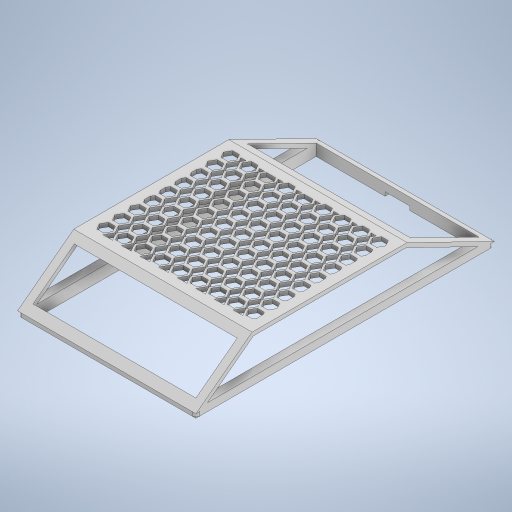
# Autodesk Inventor part: TopLid
Saved by Autodesk Inventor 2023.4 (Build 274418000, 418)
## iProperties
Created: 2026-02-22
Part Number: TopLid
Material: Generic
Document SubType Name: Modeling
Designer: 1017208
Density: 1 g/cm^3
Appearance: Default
Author: 1017208
## iProperties of the stored document TopLid_3DPrint.ipt
Created: 2026-02-22
Part Number: TopLid_3DPrint
Material: Generic
Document SubType Name: Modeling
Designer: 1017208
Density: 1 g/cm^3
Appearance: Default
Author: 1017208
Autodesk Inventor part; units mm, degrees
(part 1 of 2)
ref_plane "YZ Plane" through (0, 0, 0) normal (1, 0, 0) x (0, 1, 0)
ref_plane "XZ Plane" through (0, 0, 0) normal (0, 1, 0) x (-1, 0, 0)
ref_plane "XY Plane" through (0, 0, 0) normal (0, 0, 1) x (1, 0, 0)
sketch "Sketch1" plane through (0, 0, 0) normal (0, 1, 0) x (-1, 0, 0)
  line L0 (0, 0) -> (-139.7, 0)
  line L1 (-139.7, 0) -> (-139.7, -238.125)
  line L2 (-139.7, -238.125) -> (0, -238.125)
  line L3 (0, -238.125) -> (0, 0)
  line L4 (-3.175, -3.175) -> (-136.525, -3.175)
  line L5 (-136.525, -3.175) -> (-136.525, -234.95)
  line L6 (-136.525, -234.95) -> (-3.175, -234.95)
  line L7 (-3.175, -234.95) -> (-3.175, -3.175)
  line L8 (0, -238.125) -> (-139.7, -238.125)
  line L9 (-69.85, -238.125) -> (-69.85, -234.95)
  line L10 (-69.85, -238.125) -> (-59.69, -238.125)
  line L11 (-59.69, -238.125) -> (-80.01, -238.125)
  line L12 (-80.01, -238.125) -> (-80.01, -234.95)
  line L13 (-80.01, -234.95) -> (-59.69, -234.95)
  line L14 (-59.69, -234.95) -> (-59.69, -238.125)
  dimension "d0" = 139.7
  dimension "d1" = 238.125
  dimension "d2" = 3.175
  dimension "d3" = 10.16
  dimension "d4" = 20.32
  constraints: 30 end point, 7 equal length, 3 perpendicular, 2 horizontal, 2 midpoint, 2 point on line, 3 other
  measures "d0" distance of L2.end L1.end
  measures "d1" distance of L1.end L0.end
  measures "d2" distance between parallel lines of L3 L7
  measures "d3" distance of L9.start L10.end
  measures "d4" distance of L12.end L13.end
extrude "Extrusion1" add sketch "Sketch1" along normal blind 3.175 contours L3 L2 L14 L6 L7 L4 L5 L12 L1 L0
sketch "Sketch2" plane through (0, 3.175, 0) normal (0, 1, 0) x (1, 0, 0)
  line L0 (0, 238.125) -> (0, 0) projected
  line L1 (139.7, 238.125) -> (80.01, 238.125) projected
  line L2 (0, 0) -> (139.7, 0)
  line L3 (139.7, 0) -> (139.7, 238.125)
  line L4 (139.7, 238.125) -> (0, 238.125)
  line L5 (0, 238.125) -> (0, 0)
  line L6 (139.7, -3.175) -> (0, -3.175)
  line L7 (-3.175, 0) -> (-3.175, 238.125)
  line L8 (0, 241.3) -> (139.7, 241.3)
  line L9 (142.875, 238.125) -> (142.875, 0)
  arc A0 (0, 241.3) -> (-3.175, 238.125) centre (0, 238.125) ccw
  arc A1 (-3.175, 0) -> (0, -3.175) centre (0, 0) ccw
  arc A2 (139.7, -3.175) -> (142.875, 0) centre (139.7, 0) ccw
  arc A3 (142.875, 238.125) -> (139.7, 241.3) centre (139.7, 238.125) ccw
  dimension "d7" = 3.175
  constraints: 16 end point, 8 point on circle, 4 centre point, 4 coincident, 4 parallel, 3 tangent, 2 perpendicular, 1 horizontal
  measures "d7" distance between parallel lines of L2 L6
extrude "Extrusion2" add sketch "Sketch2" along normal blind 3.175 contours L4 L1 L3 L2 L0 | L6 A1 L7 A0 L8 A3 L9 A2
sketch "Sketch3" plane through (142.875, 3.175, 0) normal (1, 0, 0) x (0, 0, -1)
  line L0 (-3.175, 3.175) -> (241.3, 3.175)
  line L1 (0, 3.175) -> (238.125, 3.175) projected
  line L2 (119.0625, 3.175) -> (119.0625, 38.1)
  line L3 (119.0625, 38.1) -> (42.8625, 38.1)
  line L4 (119.0625, 38.1) -> (169.8625, 38.1)
  line L5 (-3.175, 3.175) -> (42.8625, 38.1)
  line L6 (169.8625, 38.1) -> (241.3, 3.175)
  line L7 (43.9305, 34.925) -> (119.0625, 34.925)
  line L8 (119.0625, 34.925) -> (169.1279, 34.925)
  line L9 (169.1279, 34.925) -> (227.5768, 6.35)
  line L10 (227.5768, 6.35) -> (6.2635, 6.35)
  line L11 (6.2635, 6.35) -> (43.9305, 34.925)
  point P0 (0, -3.175)
  dimension "d10" = 34.925
  dimension "d11" = 76.2
  dimension "d12" = 50.8
  dimension "d13" = 3.175
  constraints: 22 end point, 3 horizontal, 1 midpoint, 1 vertical, 4 other
  measures "d10" distance of L2.start L2.end
  measures "d11" distance of L2.end L3.end
  measures "d12" distance of L2.end L4.end
  measures "d13" distance between parallel lines of L3 L7
extrude "Extrusion3" add sketch "Sketch3" against normal blind 146.05 contours L5 L3 L2 L7 L11 L10 L0 | L2 L10 L9 L8 L4 L6 L0
sketch "Sketch4" plane through (0, 0, 0) normal (0, -1, 0) x (1, 0, 0)
  line L0 (0, 0) -> (139.7, 0) projected
  line L1 (0, -238.125) -> (139.7, -238.125) projected
  line L2 (0, 0) -> (139.7, 0)
  line L3 (139.7, 0) -> (139.7, -238.125)
  line L4 (139.7, -238.125) -> (0, -238.125)
  line L5 (0, -238.125) -> (0, 0)
  line L6 (136.525, -234.95) -> (136.525, -3.175)
  line L7 (136.525, -3.175) -> (3.175, -3.175)
  line L8 (3.175, -3.175) -> (3.175, -234.95)
  line L9 (3.175, -234.95) -> (136.525, -234.95)
  constraints: 16 end point, 4 parallel, 2 perpendicular, 1 horizontal, 3 other
extrude "Extrusion4" cut sketch "Sketch4" against normal blind 36.83 contours L9 L8 L7 L6
sketch "Sketch5" plane through (142.875, 41.275, -42.8625) normal (0, 1, 0) x (1, 0, 0)
  line L0 (-146.05, 127) -> (0, 127)
  line L1 (-3.6662, 6.35) -> (-149.7162, 6.35)
  line L2 (-149.7162, 6.35) -> (-146.05, 127)
  line L3 (-130.175, 122.2375) -> (-126.5088, 115.8875)
  line L4 (-126.5088, 115.8875) -> (-130.175, 109.5375)
  line L5 (-130.175, 109.5375) -> (-137.5073, 109.5375)
  line L6 (-137.5073, 109.5375) -> (-141.1735, 115.8875)
  line L7 (-141.1735, 115.8875) -> (-137.5073, 122.2375)
  line L8 (-137.5073, 122.2375) -> (-130.175, 122.2375)
  line L9 (-114.935, 122.2375) -> (-111.2688, 115.8875)
  line L10 (-111.2688, 115.8875) -> (-114.935, 109.5375)
  line L11 (-114.935, 109.5375) -> (-122.2673, 109.5375)
  line L12 (-122.2673, 109.5375) -> (-125.9335, 115.8875)
  line L13 (-125.9335, 115.8875) -> (-122.2673, 122.2375)
  line L14 (-122.2673, 122.2375) -> (-114.935, 122.2375)
  line L15 (-99.695, 122.2375) -> (-96.0288, 115.8875)
  line L16 (-96.0288, 115.8875) -> (-99.695, 109.5375)
  line L17 (-99.695, 109.5375) -> (-107.0273, 109.5375)
  line L18 (-107.0273, 109.5375) -> (-110.6935, 115.8875)
  line L19 (-110.6935, 115.8875) -> (-107.0273, 122.2375)
  line L20 (-107.0273, 122.2375) -> (-99.695, 122.2375)
  line L21 (-84.455, 122.2375) -> (-80.7888, 115.8875)
  line L22 (-80.7888, 115.8875) -> (-84.455, 109.5375)
  line L23 (-84.455, 109.5375) -> (-91.7873, 109.5375)
  line L24 (-91.7873, 109.5375) -> (-95.4535, 115.8875)
  line L25 (-95.4535, 115.8875) -> (-91.7873, 122.2375)
  line L26 (-91.7873, 122.2375) -> (-84.455, 122.2375)
  line L27 (-69.215, 122.2375) -> (-65.5488, 115.8875)
  line L28 (-65.5488, 115.8875) -> (-69.215, 109.5375)
  line L29 (-69.215, 109.5375) -> (-76.5473, 109.5375)
  line L30 (-76.5473, 109.5375) -> (-80.2135, 115.8875)
  line L31 (-80.2135, 115.8875) -> (-76.5473, 122.2375)
  line L32 (-76.5473, 122.2375) -> (-69.215, 122.2375)
  line L33 (-53.975, 122.2375) -> (-50.3088, 115.8875)
  line L34 (-50.3088, 115.8875) -> (-53.975, 109.5375)
  line L35 (-53.975, 109.5375) -> (-61.3073, 109.5375)
  line L36 (-61.3073, 109.5375) -> (-64.9735, 115.8875)
  line L37 (-64.9735, 115.8875) -> (-61.3073, 122.2375)
  line L38 (-61.3073, 122.2375) -> (-53.975, 122.2375)
  line L39 (-38.735, 122.2375) -> (-35.0688, 115.8875)
  line L40 (-35.0688, 115.8875) -> (-38.735, 109.5375)
  line L41 (-38.735, 109.5375) -> (-46.0673, 109.5375)
  line L42 (-46.0673, 109.5375) -> (-49.7335, 115.8875)
  line L43 (-49.7335, 115.8875) -> (-46.0673, 122.2375)
  line L44 (-46.0673, 122.2375) -> (-38.735, 122.2375)
  line L45 (-23.495, 122.2375) -> (-19.8288, 115.8875)
  line L46 (-19.8288, 115.8875) -> (-23.495, 109.5375)
  line L47 (-23.495, 109.5375) -> (-30.8273, 109.5375)
  line L48 (-30.8273, 109.5375) -> (-34.4935, 115.8875)
  line L49 (-34.4935, 115.8875) -> (-30.8273, 122.2375)
  line L50 (-30.8273, 122.2375) -> (-23.495, 122.2375)
  line L51 (-8.255, 122.2375) -> (-4.5888, 115.8875)
  line L52 (-4.5888, 115.8875) -> (-8.255, 109.5375)
  line L53 (-8.255, 109.5375) -> (-15.5873, 109.5375)
  line L54 (-15.5873, 109.5375) -> (-19.2535, 115.8875)
  line L55 (-19.2535, 115.8875) -> (-15.5873, 122.2375)
  line L56 (-15.5873, 122.2375) -> (-8.255, 122.2375)
  line L57 (-130.175, 109.5375) -> (-126.5088, 103.1875)
  line L58 (-126.5088, 103.1875) -> (-130.175, 96.8375)
  line L59 (-130.175, 96.8375) -> (-137.5073, 96.8375)
  line L60 (-137.5073, 96.8375) -> (-141.1735, 103.1875)
  line L61 (-141.1735, 103.1875) -> (-137.5073, 109.5375)
  line L62 (-137.5073, 109.5375) -> (-130.175, 109.5375)
  line L63 (-114.935, 109.5375) -> (-111.2688, 103.1875)
  line L64 (-111.2688, 103.1875) -> (-114.935, 96.8375)
  line L65 (-114.935, 96.8375) -> (-122.2673, 96.8375)
  line L66 (-122.2673, 96.8375) -> (-125.9335, 103.1875)
  line L67 (-125.9335, 103.1875) -> (-122.2673, 109.5375)
  line L68 (-122.2673, 109.5375) -> (-114.935, 109.5375)
  line L69 (-99.695, 109.5375) -> (-96.0288, 103.1875)
  line L70 (-96.0288, 103.1875) -> (-99.695, 96.8375)
  line L71 (-99.695, 96.8375) -> (-107.0273, 96.8375)
  line L72 (-107.0273, 96.8375) -> (-110.6935, 103.1875)
  line L73 (-110.6935, 103.1875) -> (-107.0273, 109.5375)
  line L74 (-107.0273, 109.5375) -> (-99.695, 109.5375)
  line L75 (-84.455, 109.5375) -> (-80.7888, 103.1875)
  line L76 (-80.7888, 103.1875) -> (-84.455, 96.8375)
  line L77 (-84.455, 96.8375) -> (-91.7873, 96.8375)
  line L78 (-91.7873, 96.8375) -> (-95.4535, 103.1875)
  line L79 (-95.4535, 103.1875) -> (-91.7873, 109.5375)
  line L80 (-91.7873, 109.5375) -> (-84.455, 109.5375)
  line L81 (-69.215, 109.5375) -> (-65.5488, 103.1875)
  line L82 (-65.5488, 103.1875) -> (-69.215, 96.8375)
  line L83 (-69.215, 96.8375) -> (-76.5473, 96.8375)
  line L84 (-76.5473, 96.8375) -> (-80.2135, 103.1875)
  line L85 (-80.2135, 103.1875) -> (-76.5473, 109.5375)
  line L86 (-76.5473, 109.5375) -> (-69.215, 109.5375)
  line L87 (-53.975, 109.5375) -> (-50.3088, 103.1875)
  line L88 (-50.3088, 103.1875) -> (-53.975, 96.8375)
  line L89 (-53.975, 96.8375) -> (-61.3073, 96.8375)
  line L90 (-61.3073, 96.8375) -> (-64.9735, 103.1875)
  line L91 (-64.9735, 103.1875) -> (-61.3073, 109.5375)
  line L92 (-61.3073, 109.5375) -> (-53.975, 109.5375)
  line L93 (-38.735, 109.5375) -> (-35.0688, 103.1875)
  line L94 (-35.0688, 103.1875) -> (-38.735, 96.8375)
  line L95 (-38.735, 96.8375) -> (-46.0673, 96.8375)
  line L96 (-46.0673, 96.8375) -> (-49.7335, 103.1875)
  line L97 (-49.7335, 103.1875) -> (-46.0673, 109.5375)
  line L98 (-46.0673, 109.5375) -> (-38.735, 109.5375)
  line L99 (-23.495, 109.5375) -> (-19.8288, 103.1875)
  line L100 (-19.8288, 103.1875) -> (-23.495, 96.8375)
  line L101 (-23.495, 96.8375) -> (-30.8273, 96.8375)
  line L102 (-30.8273, 96.8375) -> (-34.4935, 103.1875)
  line L103 (-34.4935, 103.1875) -> (-30.8273, 109.5375)
  line L104 (-30.8273, 109.5375) -> (-23.495, 109.5375)
  line L105 (-8.255, 109.5375) -> (-4.5888, 103.1875)
  line L106 (-4.5888, 103.1875) -> (-8.255, 96.8375)
  line L107 (-8.255, 96.8375) -> (-15.5873, 96.8375)
  line L108 (-15.5873, 96.8375) -> (-19.2535, 103.1875)
  line L109 (-19.2535, 103.1875) -> (-15.5873, 109.5375)
  line L110 (-15.5873, 109.5375) -> (-8.255, 109.5375)
  line L111 (-130.175, 96.8375) -> (-126.5088, 90.4875)
  line L112 (-126.5088, 90.4875) -> (-130.175, 84.1375)
  line L113 (-130.175, 84.1375) -> (-137.5073, 84.1375)
  line L114 (-137.5073, 84.1375) -> (-141.1735, 90.4875)
  line L115 (-141.1735, 90.4875) -> (-137.5073, 96.8375)
  line L116 (-137.5073, 96.8375) -> (-130.175, 96.8375)
  line L117 (-114.935, 96.8375) -> (-111.2688, 90.4875)
  line L118 (-111.2688, 90.4875) -> (-114.935, 84.1375)
  line L119 (-114.935, 84.1375) -> (-122.2673, 84.1375)
  line L120 (-122.2673, 84.1375) -> (-125.9335, 90.4875)
  line L121 (-125.9335, 90.4875) -> (-122.2673, 96.8375)
  line L122 (-122.2673, 96.8375) -> (-114.935, 96.8375)
  line L123 (-99.695, 96.8375) -> (-96.0288, 90.4875)
  line L124 (-96.0288, 90.4875) -> (-99.695, 84.1375)
  line L125 (-99.695, 84.1375) -> (-107.0273, 84.1375)
  line L126 (-107.0273, 84.1375) -> (-110.6935, 90.4875)
  line L127 (-110.6935, 90.4875) -> (-107.0273, 96.8375)
  line L128 (-107.0273, 96.8375) -> (-99.695, 96.8375)
  line L129 (-84.455, 96.8375) -> (-80.7888, 90.4875)
  line L130 (-80.7888, 90.4875) -> (-84.455, 84.1375)
  line L131 (-84.455, 84.1375) -> (-91.7873, 84.1375)
  line L132 (-91.7873, 84.1375) -> (-95.4535, 90.4875)
  line L133 (-95.4535, 90.4875) -> (-91.7873, 96.8375)
  line L134 (-91.7873, 96.8375) -> (-84.455, 96.8375)
  line L135 (-69.215, 96.8375) -> (-65.5488, 90.4875)
  line L136 (-65.5488, 90.4875) -> (-69.215, 84.1375)
  line L137 (-69.215, 84.1375) -> (-76.5473, 84.1375)
  line L138 (-76.5473, 84.1375) -> (-80.2135, 90.4875)
  line L139 (-80.2135, 90.4875) -> (-76.5473, 96.8375)
  line L140 (-76.5473, 96.8375) -> (-69.215, 96.8375)
  line L141 (-53.975, 96.8375) -> (-50.3088, 90.4875)
  line L142 (-50.3088, 90.4875) -> (-53.975, 84.1375)
  line L143 (-53.975, 84.1375) -> (-61.3073, 84.1375)
  line L144 (-61.3073, 84.1375) -> (-64.9735, 90.4875)
  line L145 (-64.9735, 90.4875) -> (-61.3073, 96.8375)
  line L146 (-61.3073, 96.8375) -> (-53.975, 96.8375)
  line L147 (-38.735, 96.8375) -> (-35.0688, 90.4875)
  line L148 (-35.0688, 90.4875) -> (-38.735, 84.1375)
  line L149 (-38.735, 84.1375) -> (-46.0673, 84.1375)
  line L150 (-46.0673, 84.1375) -> (-49.7335, 90.4875)
  line L151 (-49.7335, 90.4875) -> (-46.0673, 96.8375)
  line L152 (-46.0673, 96.8375) -> (-38.735, 96.8375)
  line L153 (-23.495, 96.8375) -> (-19.8288, 90.4875)
  line L154 (-19.8288, 90.4875) -> (-23.495, 84.1375)
  line L155 (-23.495, 84.1375) -> (-30.8273, 84.1375)
  line L156 (-30.8273, 84.1375) -> (-34.4935, 90.4875)
  line L157 (-34.4935, 90.4875) -> (-30.8273, 96.8375)
  line L158 (-30.8273, 96.8375) -> (-23.495, 96.8375)
  line L159 (-8.255, 96.8375) -> (-4.5888, 90.4875)
  line L160 (-4.5888, 90.4875) -> (-8.255, 84.1375)
  line L161 (-8.255, 84.1375) -> (-15.5873, 84.1375)
  line L162 (-15.5873, 84.1375) -> (-19.2535, 90.4875)
  line L163 (-19.2535, 90.4875) -> (-15.5873, 96.8375)
  line L164 (-15.5873, 96.8375) -> (-8.255, 96.8375)
  line L165 (-130.175, 84.1375) -> (-126.5088, 77.7875)
  line L166 (-126.5088, 77.7875) -> (-130.175, 71.4375)
  line L167 (-130.175, 71.4375) -> (-137.5073, 71.4375)
  line L168 (-137.5073, 71.4375) -> (-141.1735, 77.7875)
  line L169 (-141.1735, 77.7875) -> (-137.5073, 84.1375)
  line L170 (-137.5073, 84.1375) -> (-130.175, 84.1375)
  line L171 (-114.935, 84.1375) -> (-111.2688, 77.7875)
  line L172 (-111.2688, 77.7875) -> (-114.935, 71.4375)
  line L173 (-114.935, 71.4375) -> (-122.2673, 71.4375)
  line L174 (-122.2673, 71.4375) -> (-125.9335, 77.7875)
  line L175 (-125.9335, 77.7875) -> (-122.2673, 84.1375)
  line L176 (-122.2673, 84.1375) -> (-114.935, 84.1375)
  line L177 (-99.695, 84.1375) -> (-96.0288, 77.7875)
  line L178 (-96.0288, 77.7875) -> (-99.695, 71.4375)
  line L179 (-99.695, 71.4375) -> (-107.0273, 71.4375)
  line L180 (-107.0273, 71.4375) -> (-110.6935, 77.7875)
  line L181 (-110.6935, 77.7875) -> (-107.0273, 84.1375)
  line L182 (-107.0273, 84.1375) -> (-99.695, 84.1375)
  line L183 (-84.455, 84.1375) -> (-80.7888, 77.7875)
  line L184 (-80.7888, 77.7875) -> (-84.455, 71.4375)
  line L185 (-84.455, 71.4375) -> (-91.7873, 71.4375)
  line L186 (-91.7873, 71.4375) -> (-95.4535, 77.7875)
  line L187 (-95.4535, 77.7875) -> (-91.7873, 84.1375)
  line L188 (-91.7873, 84.1375) -> (-84.455, 84.1375)
  line L189 (-69.215, 84.1375) -> (-65.5488, 77.7875)
  line L190 (-65.5488, 77.7875) -> (-69.215, 71.4375)
  line L191 (-69.215, 71.4375) -> (-76.5473, 71.4375)
  line L192 (-76.5473, 71.4375) -> (-80.2135, 77.7875)
  line L193 (-80.2135, 77.7875) -> (-76.5473, 84.1375)
  line L194 (-76.5473, 84.1375) -> (-69.215, 84.1375)
  line L195 (-53.975, 84.1375) -> (-50.3088, 77.7875)
  line L196 (-50.3088, 77.7875) -> (-53.975, 71.4375)
  line L197 (-53.975, 71.4375) -> (-61.3073, 71.4375)
  line L198 (-61.3073, 71.4375) -> (-64.9735, 77.7875)
  line L199 (-64.9735, 77.7875) -> (-61.3073, 84.1375)
  line L200 (-61.3073, 84.1375) -> (-53.975, 84.1375)
  line L201 (-38.735, 84.1375) -> (-35.0688, 77.7875)
  line L202 (-35.0688, 77.7875) -> (-38.735, 71.4375)
  line L203 (-38.735, 71.4375) -> (-46.0673, 71.4375)
  line L204 (-46.0673, 71.4375) -> (-49.7335, 77.7875)
  line L205 (-49.7335, 77.7875) -> (-46.0673, 84.1375)
  line L206 (-46.0673, 84.1375) -> (-38.735, 84.1375)
  line L207 (-23.495, 84.1375) -> (-19.8288, 77.7875)
  line L208 (-19.8288, 77.7875) -> (-23.495, 71.4375)
  line L209 (-23.495, 71.4375) -> (-30.8273, 71.4375)
  line L210 (-30.8273, 71.4375) -> (-34.4935, 77.7875)
  line L211 (-34.4935, 77.7875) -> (-30.8273, 84.1375)
  line L212 (-30.8273, 84.1375) -> (-23.495, 84.1375)
  line L213 (-8.255, 84.1375) -> (-4.5888, 77.7875)
  line L214 (-4.5888, 77.7875) -> (-8.255, 71.4375)
  line L215 (-8.255, 71.4375) -> (-15.5873, 71.4375)
  line L216 (-15.5873, 71.4375) -> (-19.2535, 77.7875)
  line L217 (-19.2535, 77.7875) -> (-15.5873, 84.1375)
  line L218 (-15.5873, 84.1375) -> (-8.255, 84.1375)
  line L219 (-130.175, 71.4375) -> (-126.5088, 65.0875)
  line L220 (-126.5088, 65.0875) -> (-130.175, 58.7375)
  line L221 (-130.175, 58.7375) -> (-137.5073, 58.7375)
  line L222 (-137.5073, 58.7375) -> (-141.1735, 65.0875)
  line L223 (-141.1735, 65.0875) -> (-137.5073, 71.4375)
  line L224 (-137.5073, 71.4375) -> (-130.175, 71.4375)
  line L225 (-114.935, 71.4375) -> (-111.2688, 65.0875)
  line L226 (-111.2688, 65.0875) -> (-114.935, 58.7375)
  line L227 (-114.935, 58.7375) -> (-122.2673, 58.7375)
  line L228 (-122.2673, 58.7375) -> (-125.9335, 65.0875)
  line L229 (-125.9335, 65.0875) -> (-122.2673, 71.4375)
  line L230 (-122.2673, 71.4375) -> (-114.935, 71.4375)
  line L231 (-99.695, 71.4375) -> (-96.0288, 65.0875)
  line L232 (-96.0288, 65.0875) -> (-99.695, 58.7375)
  line L233 (-99.695, 58.7375) -> (-107.0273, 58.7375)
  line L234 (-107.0273, 58.7375) -> (-110.6935, 65.0875)
  line L235 (-110.6935, 65.0875) -> (-107.0273, 71.4375)
  line L236 (-107.0273, 71.4375) -> (-99.695, 71.4375)
  line L237 (-84.455, 71.4375) -> (-80.7888, 65.0875)
  line L238 (-80.7888, 65.0875) -> (-84.455, 58.7375)
  line L239 (-84.455, 58.7375) -> (-91.7873, 58.7375)
  line L240 (-91.7873, 58.7375) -> (-95.4535, 65.0875)
  line L241 (-95.4535, 65.0875) -> (-91.7873, 71.4375)
  line L242 (-91.7873, 71.4375) -> (-84.455, 71.4375)
  line L243 (-69.215, 71.4375) -> (-65.5488, 65.0875)
  line L244 (-65.5488, 65.0875) -> (-69.215, 58.7375)
  line L245 (-69.215, 58.7375) -> (-76.5473, 58.7375)
  line L246 (-76.5473, 58.7375) -> (-80.2135, 65.0875)
  line L247 (-80.2135, 65.0875) -> (-76.5473, 71.4375)
  line L248 (-76.5473, 71.4375) -> (-69.215, 71.4375)
  line L249 (-53.975, 71.4375) -> (-50.3088, 65.0875)
  line L250 (-50.3088, 65.0875) -> (-53.975, 58.7375)
  line L251 (-53.975, 58.7375) -> (-61.3073, 58.7375)
  line L252 (-61.3073, 58.7375) -> (-64.9735, 65.0875)
  line L253 (-64.9735, 65.0875) -> (-61.3073, 71.4375)
  line L254 (-61.3073, 71.4375) -> (-53.975, 71.4375)
  line L255 (-38.735, 71.4375) -> (-35.0688, 65.0875)
  line L256 (-35.0688, 65.0875) -> (-38.735, 58.7375)
  line L257 (-38.735, 58.7375) -> (-46.0673, 58.7375)
  line L258 (-46.0673, 58.7375) -> (-49.7335, 65.0875)
  line L259 (-49.7335, 65.0875) -> (-46.0673, 71.4375)
  line L260 (-46.0673, 71.4375) -> (-38.735, 71.4375)
  line L261 (-23.495, 71.4375) -> (-19.8288, 65.0875)
  line L262 (-19.8288, 65.0875) -> (-23.495, 58.7375)
  line L263 (-23.495, 58.7375) -> (-30.8273, 58.7375)
  line L264 (-30.8273, 58.7375) -> (-34.4935, 65.0875)
  line L265 (-34.4935, 65.0875) -> (-30.8273, 71.4375)
  line L266 (-30.8273, 71.4375) -> (-23.495, 71.4375)
  line L267 (-8.255, 71.4375) -> (-4.5888, 65.0875)
  line L268 (-4.5888, 65.0875) -> (-8.255, 58.7375)
  line L269 (-8.255, 58.7375) -> (-15.5873, 58.7375)
  line L270 (-15.5873, 58.7375) -> (-19.2535, 65.0875)
  line L271 (-19.2535, 65.0875) -> (-15.5873, 71.4375)
  line L272 (-15.5873, 71.4375) -> (-8.255, 71.4375)
  line L273 (-130.175, 58.7375) -> (-126.5088, 52.3875)
  line L274 (-126.5088, 52.3875) -> (-130.175, 46.0375)
  line L275 (-130.175, 46.0375) -> (-137.5073, 46.0375)
  line L276 (-137.5073, 46.0375) -> (-141.1735, 52.3875)
  line L277 (-141.1735, 52.3875) -> (-137.5073, 58.7375)
  line L278 (-137.5073, 58.7375) -> (-130.175, 58.7375)
  line L279 (-114.935, 58.7375) -> (-111.2688, 52.3875)
  line L280 (-111.2688, 52.3875) -> (-114.935, 46.0375)
  line L281 (-114.935, 46.0375) -> (-122.2673, 46.0375)
  line L282 (-122.2673, 46.0375) -> (-125.9335, 52.3875)
  line L283 (-125.9335, 52.3875) -> (-122.2673, 58.7375)
  line L284 (-122.2673, 58.7375) -> (-114.935, 58.7375)
  line L285 (-99.695, 58.7375) -> (-96.0288, 52.3875)
  line L286 (-96.0288, 52.3875) -> (-99.695, 46.0375)
  line L287 (-99.695, 46.0375) -> (-107.0273, 46.0375)
  line L288 (-107.0273, 46.0375) -> (-110.6935, 52.3875)
  line L289 (-110.6935, 52.3875) -> (-107.0273, 58.7375)
  line L290 (-107.0273, 58.7375) -> (-99.695, 58.7375)
  line L291 (-84.455, 58.7375) -> (-80.7888, 52.3875)
  line L292 (-80.7888, 52.3875) -> (-84.455, 46.0375)
  line L293 (-84.455, 46.0375) -> (-91.7873, 46.0375)
  line L294 (-91.7873, 46.0375) -> (-95.4535, 52.3875)
  line L295 (-95.4535, 52.3875) -> (-91.7873, 58.7375)
  line L296 (-91.7873, 58.7375) -> (-84.455, 58.7375)
  line L297 (-69.215, 58.7375) -> (-65.5488, 52.3875)
  line L298 (-65.5488, 52.3875) -> (-69.215, 46.0375)
  line L299 (-69.215, 46.0375) -> (-76.5473, 46.0375)
  line L300 (-76.5473, 46.0375) -> (-80.2135, 52.3875)
  line L301 (-80.2135, 52.3875) -> (-76.5473, 58.7375)
  line L302 (-76.5473, 58.7375) -> (-69.215, 58.7375)
  line L303 (-53.975, 58.7375) -> (-50.3088, 52.3875)
  line L304 (-50.3088, 52.3875) -> (-53.975, 46.0375)
  line L305 (-53.975, 46.0375) -> (-61.3073, 46.0375)
  line L306 (-61.3073, 46.0375) -> (-64.9735, 52.3875)
  line L307 (-64.9735, 52.3875) -> (-61.3073, 58.7375)
  line L308 (-61.3073, 58.7375) -> (-53.975, 58.7375)
  line L309 (-38.735, 58.7375) -> (-35.0688, 52.3875)
  line L310 (-35.0688, 52.3875) -> (-38.735, 46.0375)
  line L311 (-38.735, 46.0375) -> (-46.0673, 46.0375)
  line L312 (-46.0673, 46.0375) -> (-49.7335, 52.3875)
  line L313 (-49.7335, 52.3875) -> (-46.0673, 58.7375)
  line L314 (-46.0673, 58.7375) -> (-38.735, 58.7375)
  line L315 (-23.495, 58.7375) -> (-19.8288, 52.3875)
  line L316 (-19.8288, 52.3875) -> (-23.495, 46.0375)
  line L317 (-23.495, 46.0375) -> (-30.8273, 46.0375)
  line L318 (-30.8273, 46.0375) -> (-34.4935, 52.3875)
  line L319 (-34.4935, 52.3875) -> (-30.8273, 58.7375)
  line L320 (-30.8273, 58.7375) -> (-23.495, 58.7375)
  line L321 (-8.255, 58.7375) -> (-4.5888, 52.3875)
  line L322 (-4.5888, 52.3875) -> (-8.255, 46.0375)
  line L323 (-8.255, 46.0375) -> (-15.5873, 46.0375)
  line L324 (-15.5873, 46.0375) -> (-19.2535, 52.3875)
  line L325 (-19.2535, 52.3875) -> (-15.5873, 58.7375)
  line L326 (-15.5873, 58.7375) -> (-8.255, 58.7375)
  line L327 (-130.175, 46.0375) -> (-126.5088, 39.6875)
  line L328 (-126.5088, 39.6875) -> (-130.175, 33.3375)
  line L329 (-130.175, 33.3375) -> (-137.5073, 33.3375)
  line L330 (-137.5073, 33.3375) -> (-141.1735, 39.6875)
  line L331 (-141.1735, 39.6875) -> (-137.5073, 46.0375)
  line L332 (-137.5073, 46.0375) -> (-130.175, 46.0375)
  line L333 (-114.935, 46.0375) -> (-111.2688, 39.6875)
  line L334 (-111.2688, 39.6875) -> (-114.935, 33.3375)
  line L335 (-114.935, 33.3375) -> (-122.2673, 33.3375)
  line L336 (-122.2673, 33.3375) -> (-125.9335, 39.6875)
  line L337 (-125.9335, 39.6875) -> (-122.2673, 46.0375)
  line L338 (-122.2673, 46.0375) -> (-114.935, 46.0375)
  line L339 (-99.695, 46.0375) -> (-96.0288, 39.6875)
  line L340 (-96.0288, 39.6875) -> (-99.695, 33.3375)
  line L341 (-99.695, 33.3375) -> (-107.0273, 33.3375)
  line L342 (-107.0273, 33.3375) -> (-110.6935, 39.6875)
  line L343 (-110.6935, 39.6875) -> (-107.0273, 46.0375)
  line L344 (-107.0273, 46.0375) -> (-99.695, 46.0375)
  line L345 (-84.455, 46.0375) -> (-80.7888, 39.6875)
  line L346 (-80.7888, 39.6875) -> (-84.455, 33.3375)
  line L347 (-84.455, 33.3375) -> (-91.7873, 33.3375)
  line L348 (-91.7873, 33.3375) -> (-95.4535, 39.6875)
  line L349 (-95.4535, 39.6875) -> (-91.7873, 46.0375)
  line L350 (-91.7873, 46.0375) -> (-84.455, 46.0375)
  line L351 (-69.215, 46.0375) -> (-65.5488, 39.6875)
  line L352 (-65.5488, 39.6875) -> (-69.215, 33.3375)
  line L353 (-69.215, 33.3375) -> (-76.5473, 33.3375)
  line L354 (-76.5473, 33.3375) -> (-80.2135, 39.6875)
  line L355 (-80.2135, 39.6875) -> (-76.5473, 46.0375)
  line L356 (-76.5473, 46.0375) -> (-69.215, 46.0375)
  line L357 (-53.975, 46.0375) -> (-50.3088, 39.6875)
  line L358 (-50.3088, 39.6875) -> (-53.975, 33.3375)
  line L359 (-53.975, 33.3375) -> (-61.3073, 33.3375)
  line L360 (-61.3073, 33.3375) -> (-64.9735, 39.6875)
  line L361 (-64.9735, 39.6875) -> (-61.3073, 46.0375)
  line L362 (-61.3073, 46.0375) -> (-53.975, 46.0375)
  line L363 (-38.735, 46.0375) -> (-35.0688, 39.6875)
  line L364 (-35.0688, 39.6875) -> (-38.735, 33.3375)
  line L365 (-38.735, 33.3375) -> (-46.0673, 33.3375)
  line L366 (-46.0673, 33.3375) -> (-49.7335, 39.6875)
  line L367 (-49.7335, 39.6875) -> (-46.0673, 46.0375)
  line L368 (-46.0673, 46.0375) -> (-38.735, 46.0375)
  line L369 (-23.495, 46.0375) -> (-19.8288, 39.6875)
  line L370 (-19.8288, 39.6875) -> (-23.495, 33.3375)
  line L371 (-23.495, 33.3375) -> (-30.8273, 33.3375)
  line L372 (-30.8273, 33.3375) -> (-34.4935, 39.6875)
  line L373 (-34.4935, 39.6875) -> (-30.8273, 46.0375)
  line L374 (-30.8273, 46.0375) -> (-23.495, 46.0375)
  line L375 (-8.255, 46.0375) -> (-4.5888, 39.6875)
  line L376 (-4.5888, 39.6875) -> (-8.255, 33.3375)
  line L377 (-8.255, 33.3375) -> (-15.5873, 33.3375)
  line L378 (-15.5873, 33.3375) -> (-19.2535, 39.6875)
  line L379 (-19.2535, 39.6875) -> (-15.5873, 46.0375)
  line L380 (-15.5873, 46.0375) -> (-8.255, 46.0375)
  line L381 (-130.175, 33.3375) -> (-126.5088, 26.9875)
  line L382 (-126.5088, 26.9875) -> (-130.175, 20.6375)
  line L383 (-130.175, 20.6375) -> (-137.5073, 20.6375)
  line L384 (-137.5073, 20.6375) -> (-141.1735, 26.9875)
  line L385 (-141.1735, 26.9875) -> (-137.5073, 33.3375)
  line L386 (-137.5073, 33.3375) -> (-130.175, 33.3375)
  line L387 (-114.935, 33.3375) -> (-111.2688, 26.9875)
  line L388 (-111.2688, 26.9875) -> (-114.935, 20.6375)
  line L389 (-114.935, 20.6375) -> (-122.2673, 20.6375)
  line L390 (-122.2673, 20.6375) -> (-125.9335, 26.9875)
  line L391 (-125.9335, 26.9875) -> (-122.2673, 33.3375)
  line L392 (-122.2673, 33.3375) -> (-114.935, 33.3375)
  line L393 (-99.695, 33.3375) -> (-96.0288, 26.9875)
  line L394 (-96.0288, 26.9875) -> (-99.695, 20.6375)
  line L395 (-99.695, 20.6375) -> (-107.0273, 20.6375)
  line L396 (-107.0273, 20.6375) -> (-110.6935, 26.9875)
  line L397 (-110.6935, 26.9875) -> (-107.0273, 33.3375)
  line L398 (-107.0273, 33.3375) -> (-99.695, 33.3375)
  line L399 (-84.455, 33.3375) -> (-80.7888, 26.9875)
  line L400 (-80.7888, 26.9875) -> (-84.455, 20.6375)
  line L401 (-84.455, 20.6375) -> (-91.7873, 20.6375)
  line L402 (-91.7873, 20.6375) -> (-95.4535, 26.9875)
  line L403 (-95.4535, 26.9875) -> (-91.7873, 33.3375)
  line L404 (-91.7873, 33.3375) -> (-84.455, 33.3375)
  line L405 (-69.215, 33.3375) -> (-65.5488, 26.9875)
  line L406 (-65.5488, 26.9875) -> (-69.215, 20.6375)
  line L407 (-69.215, 20.6375) -> (-76.5473, 20.6375)
  line L408 (-76.5473, 20.6375) -> (-80.2135, 26.9875)
  line L409 (-80.2135, 26.9875) -> (-76.5473, 33.3375)
  line L410 (-76.5473, 33.3375) -> (-69.215, 33.3375)
  line L411 (-53.975, 33.3375) -> (-50.3088, 26.9875)
  line L412 (-50.3088, 26.9875) -> (-53.975, 20.6375)
  line L413 (-53.975, 20.6375) -> (-61.3073, 20.6375)
  line L414 (-61.3073, 20.6375) -> (-64.9735, 26.9875)
  line L415 (-64.9735, 26.9875) -> (-61.3073, 33.3375)
  line L416 (-61.3073, 33.3375) -> (-53.975, 33.3375)
  line L417 (-38.735, 33.3375) -> (-35.0688, 26.9875)
  line L418 (-35.0688, 26.9875) -> (-38.735, 20.6375)
  line L419 (-38.735, 20.6375) -> (-46.0673, 20.6375)
  line L420 (-46.0673, 20.6375) -> (-49.7335, 26.9875)
  line L421 (-49.7335, 26.9875) -> (-46.0673, 33.3375)
  line L422 (-46.0673, 33.3375) -> (-38.735, 33.3375)
  line L423 (-23.495, 33.3375) -> (-19.8288, 26.9875)
  line L424 (-19.8288, 26.9875) -> (-23.495, 20.6375)
  line L425 (-23.495, 20.6375) -> (-30.8273, 20.6375)
  line L426 (-30.8273, 20.6375) -> (-34.4935, 26.9875)
  line L427 (-34.4935, 26.9875) -> (-30.8273, 33.3375)
  line L428 (-30.8273, 33.3375) -> (-23.495, 33.3375)
  line L429 (-8.255, 33.3375) -> (-4.5888, 26.9875)
  line L430 (-4.5888, 26.9875) -> (-8.255, 20.6375)
  line L431 (-8.255, 20.6375) -> (-15.5873, 20.6375)
  line L432 (-15.5873, 20.6375) -> (-19.2535, 26.9875)
  line L433 (-19.2535, 26.9875) -> (-15.5873, 33.3375)
  line L434 (-15.5873, 33.3375) -> (-8.255, 33.3375)
  line L435 (-130.175, 20.6375) -> (-126.5088, 14.2875)
  line L436 (-126.5088, 14.2875) -> (-130.175, 7.9375)
  line L437 (-130.175, 7.9375) -> (-137.5073, 7.9375)
  line L438 (-137.5073, 7.9375) -> (-141.1735, 14.2875)
  line L439 (-141.1735, 14.2875) -> (-137.5073, 20.6375)
  line L440 (-137.5073, 20.6375) -> (-130.175, 20.6375)
  line L441 (-114.935, 20.6375) -> (-111.2688, 14.2875)
  line L442 (-111.2688, 14.2875) -> (-114.935, 7.9375)
  line L443 (-114.935, 7.9375) -> (-122.2673, 7.9375)
  line L444 (-122.2673, 7.9375) -> (-125.9335, 14.2875)
  line L445 (-125.9335, 14.2875) -> (-122.2673, 20.6375)
  line L446 (-122.2673, 20.6375) -> (-114.935, 20.6375)
  line L447 (-99.695, 20.6375) -> (-96.0288, 14.2875)
  line L448 (-96.0288, 14.2875) -> (-99.695, 7.9375)
  line L449 (-99.695, 7.9375) -> (-107.0273, 7.9375)
  line L450 (-107.0273, 7.9375) -> (-110.6935, 14.2875)
  line L451 (-110.6935, 14.2875) -> (-107.0273, 20.6375)
  line L452 (-107.0273, 20.6375) -> (-99.695, 20.6375)
  line L453 (-84.455, 20.6375) -> (-80.7888, 14.2875)
  line L454 (-80.7888, 14.2875) -> (-84.455, 7.9375)
  line L455 (-84.455, 7.9375) -> (-91.7873, 7.9375)
  line L456 (-91.7873, 7.9375) -> (-95.4535, 14.2875)
  line L457 (-95.4535, 14.2875) -> (-91.7873, 20.6375)
  line L458 (-91.7873, 20.6375) -> (-84.455, 20.6375)
  line L459 (-69.215, 20.6375) -> (-65.5488, 14.2875)
  line L460 (-65.5488, 14.2875) -> (-69.215, 7.9375)
  line L461 (-69.215, 7.9375) -> (-76.5473, 7.9375)
  line L462 (-76.5473, 7.9375) -> (-80.2135, 14.2875)
  line L463 (-80.2135, 14.2875) -> (-76.5473, 20.6375)
  line L464 (-76.5473, 20.6375) -> (-69.215, 20.6375)
  line L465 (-53.975, 20.6375) -> (-50.3088, 14.2875)
  line L466 (-50.3088, 14.2875) -> (-53.975, 7.9375)
  line L467 (-53.975, 7.9375) -> (-61.3073, 7.9375)
  line L468 (-61.3073, 7.9375) -> (-64.9735, 14.2875)
  line L469 (-64.9735, 14.2875) -> (-61.3073, 20.6375)
  line L470 (-61.3073, 20.6375) -> (-53.975, 20.6375)
  line L471 (-38.735, 20.6375) -> (-35.0688, 14.2875)
  line L472 (-35.0688, 14.2875) -> (-38.735, 7.9375)
  line L473 (-38.735, 7.9375) -> (-46.0673, 7.9375)
  line L474 (-46.0673, 7.9375) -> (-49.7335, 14.2875)
  line L475 (-49.7335, 14.2875) -> (-46.0673, 20.6375)
  line L476 (-46.0673, 20.6375) -> (-38.735, 20.6375)
  line L477 (-23.495, 20.6375) -> (-19.8288, 14.2875)
  line L478 (-19.8288, 14.2875) -> (-23.495, 7.9375)
  line L479 (-23.495, 7.9375) -> (-30.8273, 7.9375)
  line L480 (-30.8273, 7.9375) -> (-34.4935, 14.2875)
  line L481 (-34.4935, 14.2875) -> (-30.8273, 20.6375)
  line L482 (-30.8273, 20.6375) -> (-23.495, 20.6375)
  line L483 (-8.255, 20.6375) -> (-4.5888, 14.2875)
  line L484 (-4.5888, 14.2875) -> (-8.255, 7.9375)
  line L485 (-8.255, 7.9375) -> (-15.5873, 7.9375)
  line L486 (-15.5873, 7.9375) -> (-19.2535, 14.2875)
  line L487 (-19.2535, 14.2875) -> (-15.5873, 20.6375)
  line L488 (-15.5873, 20.6375) -> (-8.255, 20.6375)
  line L489 (-146.05, 1.068) -> (-146.05, -36.599) projected
  line L490 (-146.05, 0) -> (0, 0)
  line L491 (0, 0) -> (0, 127)
  line L492 (0, 127) -> (-146.05, 127)
  line L493 (-146.05, 127) -> (-146.05, 0)
  line L494 (-7.9375, 7.9375) -> (-138.1125, 7.9375)
  line L495 (-138.1125, 7.9375) -> (-138.1125, 119.0625)
  line L496 (-138.1125, 119.0625) -> (-7.9375, 119.0625)
  line L497 (-7.9375, 119.0625) -> (-7.9375, 7.9375)
  line L498 (-131.0915, 111.125) -> (-128.3419, 115.8875)
  line L499 (-128.3419, 115.8875) -> (-131.0915, 120.65)
  line L500 (-131.0915, 120.65) -> (-136.5908, 120.65)
  line L501 (-136.5908, 120.65) -> (-139.3404, 115.8875)
  line L502 (-139.3404, 115.8875) -> (-136.5908, 111.125)
  line L503 (-136.5908, 111.125) -> (-131.0915, 111.125)
  line L504 (-131.0915, 107.95) -> (-136.5908, 107.95)
  line L505 (-136.5908, 107.95) -> (-139.3404, 103.1875)
  line L506 (-128.3419, 103.1875) -> (-131.0915, 107.95)
  line L507 (-131.0915, 98.425) -> (-128.3419, 103.1875)
  line L508 (-136.5908, 98.425) -> (-131.0915, 98.425)
  line L509 (-139.3404, 103.1875) -> (-136.5908, 98.425)
  line L510 (-131.0915, 95.25) -> (-136.5908, 95.25)
  line L511 (-136.5908, 95.25) -> (-139.3404, 90.4875)
  line L512 (-128.3419, 90.4875) -> (-131.0915, 95.25)
  line L513 (-131.0915, 85.725) -> (-128.3419, 90.4875)
  line L514 (-136.5908, 85.725) -> (-131.0915, 85.725)
  line L515 (-139.3404, 90.4875) -> (-136.5908, 85.725)
  line L516 (-131.0915, 82.55) -> (-136.5908, 82.55)
  line L517 (-136.5908, 82.55) -> (-139.3404, 77.7875)
  line L518 (-128.3419, 77.7875) -> (-131.0915, 82.55)
  line L519 (-131.0915, 73.025) -> (-128.3419, 77.7875)
  line L520 (-136.5908, 73.025) -> (-131.0915, 73.025)
  line L521 (-139.3404, 77.7875) -> (-136.5908, 73.025)
  line L522 (-131.0915, 69.85) -> (-136.5908, 69.85)
  line L523 (-136.5908, 69.85) -> (-139.3404, 65.0875)
  line L524 (-128.3419, 65.0875) -> (-131.0915, 69.85)
  line L525 (-131.0915, 60.325) -> (-128.3419, 65.0875)
  line L526 (-136.5908, 60.325) -> (-131.0915, 60.325)
  line L527 (-139.3404, 65.0875) -> (-136.5908, 60.325)
  line L528 (-131.0915, 57.15) -> (-136.5908, 57.15)
  line L529 (-136.5908, 57.15) -> (-139.3404, 52.3875)
  line L530 (-128.3419, 52.3875) -> (-131.0915, 57.15)
  line L531 (-131.0915, 47.625) -> (-128.3419, 52.3875)
  line L532 (-136.5908, 47.625) -> (-131.0915, 47.625)
  line L533 (-139.3404, 52.3875) -> (-136.5908, 47.625)
  line L534 (-131.0915, 44.45) -> (-136.5908, 44.45)
  line L535 (-136.5908, 44.45) -> (-139.3404, 39.6875)
  line L536 (-128.3419, 39.6875) -> (-131.0915, 44.45)
  line L537 (-131.0915, 34.925) -> (-128.3419, 39.6875)
  line L538 (-136.5908, 34.925) -> (-131.0915, 34.925)
  line L539 (-139.3404, 39.6875) -> (-136.5908, 34.925)
  line L540 (-131.0915, 31.75) -> (-136.5908, 31.75)
  line L541 (-136.5908, 31.75) -> (-139.3404, 26.9875)
  line L542 (-128.3419, 26.9875) -> (-131.0915, 31.75)
  line L543 (-131.0915, 22.225) -> (-128.3419, 26.9875)
  line L544 (-136.5908, 22.225) -> (-131.0915, 22.225)
  line L545 (-139.3404, 26.9875) -> (-136.5908, 22.225)
  line L546 (-131.0915, 19.05) -> (-136.5908, 19.05)
  line L547 (-136.5908, 19.05) -> (-139.3404, 14.2875)
  line L548 (-128.3419, 14.2875) -> (-131.0915, 19.05)
  line L549 (-131.0915, 9.525) -> (-128.3419, 14.2875)
  line L550 (-136.5908, 9.525) -> (-131.0915, 9.525)
  line L551 (-139.3404, 14.2875) -> (-136.5908, 9.525)
  line L552 (-115.8515, 120.65) -> (-121.3508, 120.65)
  line L553 (-121.3508, 120.65) -> (-124.1004, 115.8875)
  line L554 (-113.1019, 115.8875) -> (-115.8515, 120.65)
  line L555 (-115.8515, 111.125) -> (-113.1019, 115.8875)
  line L556 (-121.3508, 111.125) -> (-115.8515, 111.125)
  line L557 (-124.1004, 115.8875) -> (-121.3508, 111.125)
  line L558 (-115.8515, 107.95) -> (-121.3508, 107.95)
  line L559 (-121.3508, 107.95) -> (-124.1004, 103.1875)
  line L560 (-113.1019, 103.1875) -> (-115.8515, 107.95)
  line L561 (-115.8515, 98.425) -> (-113.1019, 103.1875)
  line L562 (-121.3508, 98.425) -> (-115.8515, 98.425)
  line L563 (-124.1004, 103.1875) -> (-121.3508, 98.425)
  line L564 (-115.8515, 95.25) -> (-121.3508, 95.25)
  line L565 (-121.3508, 95.25) -> (-124.1004, 90.4875)
  line L566 (-113.1019, 90.4875) -> (-115.8515, 95.25)
  line L567 (-115.8515, 85.725) -> (-113.1019, 90.4875)
  line L568 (-121.3508, 85.725) -> (-115.8515, 85.725)
  line L569 (-124.1004, 90.4875) -> (-121.3508, 85.725)
  line L570 (-115.8515, 82.55) -> (-121.3508, 82.55)
  line L571 (-121.3508, 82.55) -> (-124.1004, 77.7875)
  line L572 (-113.1019, 77.7875) -> (-115.8515, 82.55)
  line L573 (-115.8515, 73.025) -> (-113.1019, 77.7875)
  line L574 (-121.3508, 73.025) -> (-115.8515, 73.025)
  line L575 (-124.1004, 77.7875) -> (-121.3508, 73.025)
  line L576 (-115.8515, 69.85) -> (-121.3508, 69.85)
  line L577 (-121.3508, 69.85) -> (-124.1004, 65.0875)
  line L578 (-113.1019, 65.0875) -> (-115.8515, 69.85)
  line L579 (-115.8515, 60.325) -> (-113.1019, 65.0875)
  line L580 (-121.3508, 60.325) -> (-115.8515, 60.325)
  line L581 (-124.1004, 65.0875) -> (-121.3508, 60.325)
  line L582 (-115.8515, 57.15) -> (-121.3508, 57.15)
  line L583 (-121.3508, 57.15) -> (-124.1004, 52.3875)
  line L584 (-113.1019, 52.3875) -> (-115.8515, 57.15)
  line L585 (-115.8515, 47.625) -> (-113.1019, 52.3875)
  line L586 (-121.3508, 47.625) -> (-115.8515, 47.625)
  line L587 (-124.1004, 52.3875) -> (-121.3508, 47.625)
  line L588 (-115.8515, 44.45) -> (-121.3508, 44.45)
  line L589 (-121.3508, 44.45) -> (-124.1004, 39.6875)
  line L590 (-113.1019, 39.6875) -> (-115.8515, 44.45)
  line L591 (-115.8515, 34.925) -> (-113.1019, 39.6875)
  line L592 (-121.3508, 34.925) -> (-115.8515, 34.925)
  line L593 (-124.1004, 39.6875) -> (-121.3508, 34.925)
  line L594 (-115.8515, 31.75) -> (-121.3508, 31.75)
  line L595 (-121.3508, 31.75) -> (-124.1004, 26.9875)
  line L596 (-113.1019, 26.9875) -> (-115.8515, 31.75)
  line L597 (-115.8515, 22.225) -> (-113.1019, 26.9875)
  line L598 (-121.3508, 22.225) -> (-115.8515, 22.225)
  line L599 (-124.1004, 26.9875) -> (-121.3508, 22.225)
  line L600 (-115.8515, 19.05) -> (-121.3508, 19.05)
  line L601 (-121.3508, 19.05) -> (-124.1004, 14.2875)
  line L602 (-113.1019, 14.2875) -> (-115.8515, 19.05)
  line L603 (-115.8515, 9.525) -> (-113.1019, 14.2875)
  line L604 (-121.3508, 9.525) -> (-115.8515, 9.525)
  line L605 (-124.1004, 14.2875) -> (-121.3508, 9.525)
  line L606 (-100.6115, 120.65) -> (-106.1108, 120.65)
  line L607 (-106.1108, 120.65) -> (-108.8604, 115.8875)
  line L608 (-97.8619, 115.8875) -> (-100.6115, 120.65)
  line L609 (-100.6115, 111.125) -> (-97.8619, 115.8875)
  line L610 (-106.1108, 111.125) -> (-100.6115, 111.125)
  line L611 (-108.8604, 115.8875) -> (-106.1108, 111.125)
  line L612 (-100.6115, 107.95) -> (-106.1108, 107.95)
  line L613 (-106.1108, 107.95) -> (-108.8604, 103.1875)
  line L614 (-97.8619, 103.1875) -> (-100.6115, 107.95)
  line L615 (-100.6115, 98.425) -> (-97.8619, 103.1875)
  line L616 (-106.1108, 98.425) -> (-100.6115, 98.425)
  line L617 (-108.8604, 103.1875) -> (-106.1108, 98.425)
  line L618 (-100.6115, 95.25) -> (-106.1108, 95.25)
  line L619 (-106.1108, 95.25) -> (-108.8604, 90.4875)
  line L620 (-97.8619, 90.4875) -> (-100.6115, 95.25)
  line L621 (-100.6115, 85.725) -> (-97.8619, 90.4875)
  line L622 (-106.1108, 85.725) -> (-100.6115, 85.725)
  line L623 (-108.8604, 90.4875) -> (-106.1108, 85.725)
  line L624 (-100.6115, 82.55) -> (-106.1108, 82.55)
  line L625 (-106.1108, 82.55) -> (-108.8604, 77.7875)
  line L626 (-97.8619, 77.7875) -> (-100.6115, 82.55)
  line L627 (-100.6115, 73.025) -> (-97.8619, 77.7875)
  line L628 (-106.1108, 73.025) -> (-100.6115, 73.025)
  line L629 (-108.8604, 77.7875) -> (-106.1108, 73.025)
  line L630 (-100.6115, 69.85) -> (-106.1108, 69.85)
  line L631 (-106.1108, 69.85) -> (-108.8604, 65.0875)
  line L632 (-97.8619, 65.0875) -> (-100.6115, 69.85)
  line L633 (-100.6115, 60.325) -> (-97.8619, 65.0875)
  line L634 (-106.1108, 60.325) -> (-100.6115, 60.325)
  line L635 (-108.8604, 65.0875) -> (-106.1108, 60.325)
  line L636 (-100.6115, 57.15) -> (-106.1108, 57.15)
  line L637 (-106.1108, 57.15) -> (-108.8604, 52.3875)
  line L638 (-97.8619, 52.3875) -> (-100.6115, 57.15)
  line L639 (-100.6115, 47.625) -> (-97.8619, 52.3875)
  line L640 (-106.1108, 47.625) -> (-100.6115, 47.625)
  line L641 (-108.8604, 52.3875) -> (-106.1108, 47.625)
  line L642 (-100.6115, 44.45) -> (-106.1108, 44.45)
  line L643 (-106.1108, 44.45) -> (-108.8604, 39.6875)
  line L644 (-97.8619, 39.6875) -> (-100.6115, 44.45)
  line L645 (-100.6115, 34.925) -> (-97.8619, 39.6875)
  line L646 (-106.1108, 34.925) -> (-100.6115, 34.925)
  line L647 (-108.8604, 39.6875) -> (-106.1108, 34.925)
  line L648 (-100.6115, 31.75) -> (-106.1108, 31.75)
  line L649 (-106.1108, 31.75) -> (-108.8604, 26.9875)
  line L650 (-97.8619, 26.9875) -> (-100.6115, 31.75)
  line L651 (-100.6115, 22.225) -> (-97.8619, 26.9875)
  line L652 (-106.1108, 22.225) -> (-100.6115, 22.225)
  line L653 (-108.8604, 26.9875) -> (-106.1108, 22.225)
  line L654 (-100.6115, 19.05) -> (-106.1108, 19.05)
  line L655 (-106.1108, 19.05) -> (-108.8604, 14.2875)
  line L656 (-97.8619, 14.2875) -> (-100.6115, 19.05)
  line L657 (-100.6115, 9.525) -> (-97.8619, 14.2875)
  line L658 (-106.1108, 9.525) -> (-100.6115, 9.525)
  line L659 (-108.8604, 14.2875) -> (-106.1108, 9.525)
  line L660 (-85.3715, 120.65) -> (-90.8708, 120.65)
  line L661 (-90.8708, 120.65) -> (-93.6204, 115.8875)
  line L662 (-82.6219, 115.8875) -> (-85.3715, 120.65)
  line L663 (-85.3715, 111.125) -> (-82.6219, 115.8875)
  line L664 (-90.8708, 111.125) -> (-85.3715, 111.125)
  line L665 (-93.6204, 115.8875) -> (-90.8708, 111.125)
  line L666 (-85.3715, 107.95) -> (-90.8708, 107.95)
  line L667 (-90.8708, 107.95) -> (-93.6204, 103.1875)
  line L668 (-82.6219, 103.1875) -> (-85.3715, 107.95)
  line L669 (-85.3715, 98.425) -> (-82.6219, 103.1875)
  line L670 (-90.8708, 98.425) -> (-85.3715, 98.425)
  line L671 (-93.6204, 103.1875) -> (-90.8708, 98.425)
  line L672 (-85.3715, 95.25) -> (-90.8708, 95.25)
  line L673 (-90.8708, 95.25) -> (-93.6204, 90.4875)
  line L674 (-82.6219, 90.4875) -> (-85.3715, 95.25)
  line L675 (-85.3715, 85.725) -> (-82.6219, 90.4875)
  line L676 (-90.8708, 85.725) -> (-85.3715, 85.725)
  line L677 (-93.6204, 90.4875) -> (-90.8708, 85.725)
  line L678 (-85.3715, 82.55) -> (-90.8708, 82.55)
  line L679 (-90.8708, 82.55) -> (-93.6204, 77.7875)
  line L680 (-82.6219, 77.7875) -> (-85.3715, 82.55)
  line L681 (-85.3715, 73.025) -> (-82.6219, 77.7875)
  line L682 (-90.8708, 73.025) -> (-85.3715, 73.025)
  line L683 (-93.6204, 77.7875) -> (-90.8708, 73.025)
  line L684 (-85.3715, 69.85) -> (-90.8708, 69.85)
  line L685 (-90.8708, 69.85) -> (-93.6204, 65.0875)
  line L686 (-82.6219, 65.0875) -> (-85.3715, 69.85)
  line L687 (-85.3715, 60.325) -> (-82.6219, 65.0875)
  line L688 (-90.8708, 60.325) -> (-85.3715, 60.325)
  line L689 (-93.6204, 65.0875) -> (-90.8708, 60.325)
  line L690 (-85.3715, 57.15) -> (-90.8708, 57.15)
  line L691 (-90.8708, 57.15) -> (-93.6204, 52.3875)
  line L692 (-82.6219, 52.3875) -> (-85.3715, 57.15)
  line L693 (-85.3715, 47.625) -> (-82.6219, 52.3875)
  line L694 (-90.8708, 47.625) -> (-85.3715, 47.625)
  line L695 (-93.6204, 52.3875) -> (-90.8708, 47.625)
  line L696 (-85.3715, 44.45) -> (-90.8708, 44.45)
  line L697 (-90.8708, 44.45) -> (-93.6204, 39.6875)
  line L698 (-82.6219, 39.6875) -> (-85.3715, 44.45)
  line L699 (-85.3715, 34.925) -> (-82.6219, 39.6875)
  line L700 (-90.8708, 34.925) -> (-85.3715, 34.925)
  line L701 (-93.6204, 39.6875) -> (-90.8708, 34.925)
  line L702 (-85.3715, 31.75) -> (-90.8708, 31.75)
  line L703 (-90.8708, 31.75) -> (-93.6204, 26.9875)
  line L704 (-82.6219, 26.9875) -> (-85.3715, 31.75)
  line L705 (-85.3715, 22.225) -> (-82.6219, 26.9875)
  line L706 (-90.8708, 22.225) -> (-85.3715, 22.225)
  line L707 (-93.6204, 26.9875) -> (-90.8708, 22.225)
  line L708 (-85.3715, 19.05) -> (-90.8708, 19.05)
  line L709 (-90.8708, 19.05) -> (-93.6204, 14.2875)
  line L710 (-82.6219, 14.2875) -> (-85.3715, 19.05)
  line L711 (-85.3715, 9.525) -> (-82.6219, 14.2875)
  line L712 (-90.8708, 9.525) -> (-85.3715, 9.525)
  line L713 (-93.6204, 14.2875) -> (-90.8708, 9.525)
  line L714 (-70.1315, 120.65) -> (-75.6308, 120.65)
  line L715 (-75.6308, 120.65) -> (-78.3804, 115.8875)
  line L716 (-67.3819, 115.8875) -> (-70.1315, 120.65)
  line L717 (-70.1315, 111.125) -> (-67.3819, 115.8875)
  line L718 (-75.6308, 111.125) -> (-70.1315, 111.125)
  line L719 (-78.3804, 115.8875) -> (-75.6308, 111.125)
  line L720 (-70.1315, 107.95) -> (-75.6308, 107.95)
  line L721 (-75.6308, 107.95) -> (-78.3804, 103.1875)
  line L722 (-67.3819, 103.1875) -> (-70.1315, 107.95)
  line L723 (-70.1315, 98.425) -> (-67.3819, 103.1875)
  line L724 (-75.6308, 98.425) -> (-70.1315, 98.425)
  line L725 (-78.3804, 103.1875) -> (-75.6308, 98.425)
  line L726 (-70.1315, 95.25) -> (-75.6308, 95.25)
  line L727 (-75.6308, 95.25) -> (-78.3804, 90.4875)
  line L728 (-67.3819, 90.4875) -> (-70.1315, 95.25)
  line L729 (-70.1315, 85.725) -> (-67.3819, 90.4875)
  line L730 (-75.6308, 85.725) -> (-70.1315, 85.725)
  line L731 (-78.3804, 90.4875) -> (-75.6308, 85.725)
  line L732 (-70.1315, 82.55) -> (-75.6308, 82.55)
  line L733 (-75.6308, 82.55) -> (-78.3804, 77.7875)
  line L734 (-67.3819, 77.7875) -> (-70.1315, 82.55)
  line L735 (-70.1315, 73.025) -> (-67.3819, 77.7875)
  line L736 (-75.6308, 73.025) -> (-70.1315, 73.025)
  line L737 (-78.3804, 77.7875) -> (-75.6308, 73.025)
  line L738 (-70.1315, 69.85) -> (-75.6308, 69.85)
  line L739 (-75.6308, 69.85) -> (-78.3804, 65.0875)
  line L740 (-67.3819, 65.0875) -> (-70.1315, 69.85)
  line L741 (-70.1315, 60.325) -> (-67.3819, 65.0875)
  line L742 (-75.6308, 60.325) -> (-70.1315, 60.325)
  line L743 (-78.3804, 65.0875) -> (-75.6308, 60.325)
  line L744 (-70.1315, 57.15) -> (-75.6308, 57.15)
  line L745 (-75.6308, 57.15) -> (-78.3804, 52.3875)
  line L746 (-67.3819, 52.3875) -> (-70.1315, 57.15)
  line L747 (-70.1315, 47.625) -> (-67.3819, 52.3875)
  line L748 (-75.6308, 47.625) -> (-70.1315, 47.625)
  line L749 (-78.3804, 52.3875) -> (-75.6308, 47.625)
  line L750 (-70.1315, 44.45) -> (-75.6308, 44.45)
  line L751 (-75.6308, 44.45) -> (-78.3804, 39.6875)
  line L752 (-67.3819, 39.6875) -> (-70.1315, 44.45)
  line L753 (-70.1315, 34.925) -> (-67.3819, 39.6875)
  line L754 (-75.6308, 34.925) -> (-70.1315, 34.925)
  line L755 (-78.3804, 39.6875) -> (-75.6308, 34.925)
  line L756 (-70.1315, 31.75) -> (-75.6308, 31.75)
  line L757 (-75.6308, 31.75) -> (-78.3804, 26.9875)
  line L758 (-67.3819, 26.9875) -> (-70.1315, 31.75)
  line L759 (-70.1315, 22.225) -> (-67.3819, 26.9875)
  line L760 (-75.6308, 22.225) -> (-70.1315, 22.225)
  line L761 (-78.3804, 26.9875) -> (-75.6308, 22.225)
  line L762 (-70.1315, 19.05) -> (-75.6308, 19.05)
  line L763 (-75.6308, 19.05) -> (-78.3804, 14.2875)
  line L764 (-67.3819, 14.2875) -> (-70.1315, 19.05)
  line L765 (-70.1315, 9.525) -> (-67.3819, 14.2875)
  line L766 (-75.6308, 9.525) -> (-70.1315, 9.525)
  line L767 (-78.3804, 14.2875) -> (-75.6308, 9.525)
  line L768 (-54.8915, 120.65) -> (-60.3908, 120.65)
  line L769 (-60.3908, 120.65) -> (-63.1404, 115.8875)
  line L770 (-52.1419, 115.8875) -> (-54.8915, 120.65)
  line L771 (-54.8915, 111.125) -> (-52.1419, 115.8875)
  line L772 (-60.3908, 111.125) -> (-54.8915, 111.125)
  line L773 (-63.1404, 115.8875) -> (-60.3908, 111.125)
  line L774 (-54.8915, 107.95) -> (-60.3908, 107.95)
  line L775 (-60.3908, 107.95) -> (-63.1404, 103.1875)
  line L776 (-52.1419, 103.1875) -> (-54.8915, 107.95)
  line L777 (-54.8915, 98.425) -> (-52.1419, 103.1875)
  line L778 (-60.3908, 98.425) -> (-54.8915, 98.425)
  line L779 (-63.1404, 103.1875) -> (-60.3908, 98.425)
  line L780 (-54.8915, 95.25) -> (-60.3908, 95.25)
  line L781 (-60.3908, 95.25) -> (-63.1404, 90.4875)
  line L782 (-52.1419, 90.4875) -> (-54.8915, 95.25)
  line L783 (-54.8915, 85.725) -> (-52.1419, 90.4875)
  line L784 (-60.3908, 85.725) -> (-54.8915, 85.725)
  line L785 (-63.1404, 90.4875) -> (-60.3908, 85.725)
  line L786 (-54.8915, 82.55) -> (-60.3908, 82.55)
  line L787 (-60.3908, 82.55) -> (-63.1404, 77.7875)
  line L788 (-52.1419, 77.7875) -> (-54.8915, 82.55)
  line L789 (-54.8915, 73.025) -> (-52.1419, 77.7875)
  line L790 (-60.3908, 73.025) -> (-54.8915, 73.025)
  line L791 (-63.1404, 77.7875) -> (-60.3908, 73.025)
  line L792 (-54.8915, 69.85) -> (-60.3908, 69.85)
  line L793 (-60.3908, 69.85) -> (-63.1404, 65.0875)
  line L794 (-52.1419, 65.0875) -> (-54.8915, 69.85)
  line L795 (-54.8915, 60.325) -> (-52.1419, 65.0875)
  line L796 (-60.3908, 60.325) -> (-54.8915, 60.325)
  line L797 (-63.1404, 65.0875) -> (-60.3908, 60.325)
  line L798 (-54.8915, 57.15) -> (-60.3908, 57.15)
  line L799 (-60.3908, 57.15) -> (-63.1404, 52.3875)
  line L800 (-52.1419, 52.3875) -> (-54.8915, 57.15)
  line L801 (-54.8915, 47.625) -> (-52.1419, 52.3875)
  line L802 (-60.3908, 47.625) -> (-54.8915, 47.625)
  line L803 (-63.1404, 52.3875) -> (-60.3908, 47.625)
  line L804 (-54.8915, 44.45) -> (-60.3908, 44.45)
  line L805 (-60.3908, 44.45) -> (-63.1404, 39.6875)
  line L806 (-52.1419, 39.6875) -> (-54.8915, 44.45)
  line L807 (-54.8915, 34.925) -> (-52.1419, 39.6875)
  line L808 (-60.3908, 34.925) -> (-54.8915, 34.925)
  line L809 (-63.1404, 39.6875) -> (-60.3908, 34.925)
  line L810 (-54.8915, 31.75) -> (-60.3908, 31.75)
  line L811 (-60.3908, 31.75) -> (-63.1404, 26.9875)
  line L812 (-52.1419, 26.9875) -> (-54.8915, 31.75)
  line L813 (-54.8915, 22.225) -> (-52.1419, 26.9875)
  line L814 (-60.3908, 22.225) -> (-54.8915, 22.225)
  line L815 (-63.1404, 26.9875) -> (-60.3908, 22.225)
  line L816 (-54.8915, 19.05) -> (-60.3908, 19.05)
  line L817 (-60.3908, 19.05) -> (-63.1404, 14.2875)
  line L818 (-52.1419, 14.2875) -> (-54.8915, 19.05)
  line L819 (-54.8915, 9.525) -> (-52.1419, 14.2875)
  line L820 (-60.3908, 9.525) -> (-54.8915, 9.525)
  line L821 (-63.1404, 14.2875) -> (-60.3908, 9.525)
  line L822 (-39.6515, 120.65) -> (-45.1508, 120.65)